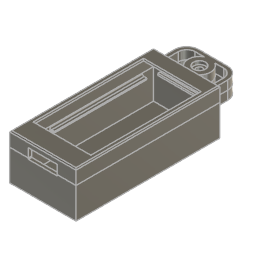
FlightSensorbyLimitens (Autodesk Fusion 360 design; units mm, degrees)
part number: 2026-05-18-21-55-51-119
Autodesk Fusion 360 part; units mm, degrees
sketch "Sketch1" plane through (0, 0, 0) normal (0, 0, 1) x (1, 0, 0)
  line L0 (-1, 32) -> (28, 32)
  line L1 (28, 32) -> (28, -31)
  line L2 (28, -31) -> (-1, -31)
  line L3 (-1, -31) -> (-1, 32)
  line L4 (30, -32) -> (-3, -32)
  line L5 (-3, -32) -> (-3, 34)
  line L6 (-3, 34) -> (30, 34)
  line L7 (30, 34) -> (30, -32)
  line L8 (21, -32) -> (6, -32)
  line L9 (6, -32) -> (6, -31)
  line L10 (6, -31) -> (21, -31)
  line L11 (21, -31) -> (21, -32)
  line L12 (21, -32) -> (6, -31) construction
  line L13 (6, -32) -> (21, -31) construction
  line L14 (19.5, -32) -> (7.5, -32)
  line L15 (7.5, -32) -> (7.5, -31)
  line L16 (7.5, -31) -> (19.5, -31)
  line L17 (19.5, -31) -> (19.5, -32)
  line L18 (19.5, -32) -> (7.5, -31) construction
  line L19 (7.5, -32) -> (19.5, -31) construction
  point P0 (13.5, -31.5)
  point P1 (13.5, -31.5)
  constraint horizontal L0
  constraint vertical L1
  constraint horizontal L2
  constraint vertical L3
  constraint horizontal L4
  constraint vertical L5
  constraint horizontal L6
  constraint vertical L7
  constraint horizontal L8
  constraint perpendicular L8 L9
  constraint parallel L8 L10
  constraint parallel L9 L11
  constraint coincident L12 P1
  constraint coincident L13 P1
  constraint coincident L4 L8.start
  constraint horizontal L14
  constraint perpendicular L14 L15
  constraint parallel L14 L16
  constraint parallel L15 L17
  constraint coincident L18 P1
  constraint coincident L19 P1
  constraint coincident L8 L14.start
  constraint coincident P1 P0
sketch "Sketch2" plane through (7.5, 0, 0) normal (1, 0, 0) x (0, 1, 0)
  line L0 (-33, -3) -> (-33, -5.5)
  line L1 (-33, -5.5) -> (-32, -5.5)
  line L2 (-31, -1.5) -> (-33, -1.5)
  line L3 (-33, -1.5) -> (-33, -5.5)
  line L4 (-33, -5.5) -> (-31, -5.5)
  line L5 (-31, -5.5) -> (-31, -1.5)
  line L6 (-32, -3) -> (-33, -3)
  line L7 (-32, -5.5) -> (-32, -3)
  constraint horizontal L2
  constraint vertical L3
  constraint horizontal L4
  constraint vertical L5
  constraint coincident L0.end L1.start
sketch "Sketch3" plane through (-1, 0, 0) normal (1, 0, 0) x (0, 1, 0)
  line L0 (32, 4) -> (-31, 4)
  line L1 (-31, -3) -> (32, -3)
  line L2 (32, -3) -> (32, 2)
  line L3 (32, 2) -> (-31, 2)
  line L4 (-31, 2) -> (-31, -3)
  line L5 (-31, 3) -> (32, 3)
  line L6 (32, 3) -> (32, 4)
  line L7 (-31, 4) -> (-31, 3)
  constraint horizontal L1
  constraint vertical L2
  constraint horizontal L3
  constraint vertical L4
sketch "Sketch4" plane through (0, 34, 0) normal (0, 1, 0) x (-1, 0, 0)
  line L0 (3, 4) -> (-30, 4)
  line L1 (-2.5, -2.5) -> (-24.5, -2.5)
  line L2 (-24.5, -2.5) -> (-24.5, 1)
  line L3 (-24.5, 1) -> (-2.5, 1)
  line L4 (-2.5, 1) -> (-2.5, -2.5)
  line L5 (-2.5, -2.5) -> (-24.5, 1) construction
  line L6 (-24.5, -2.5) -> (-2.5, 1) construction
  line L7 (3, 3) -> (3, 4)
  line L8 (-30, 4) -> (-30, 3)
  line L9 (-30, 3) -> (3, 3)
  point P0 (-13.5, -0.75)
  constraint horizontal L1
  constraint perpendicular L1 L2
  constraint parallel L1 L3
  constraint parallel L2 L4
  constraint coincident L5 P0
  constraint coincident L6 P0
ref_plane "WorkPlane1" through (13.5, -32, -0.5) normal (0, 0, -1) x (-1, 0, 0)
sketch "Sketch5" plane through (0, 0, 3) normal (0, 0, 1) x (-1, 0, 0)
  circle A0 centre (-13.5, -37.8128) radius 2.75
  arc A1 (-7.5, -42) -> (-2.5, -37) centre (-7.5, -37) ccw
  line L0 (-2.5, -37) -> (-2.5, -34)
  line L1 (-24.5, -34) -> (-24.5, -37)
  arc A2 (-24.5, -37) -> (-19.5, -42) centre (-19.5, -37) ccw
  line L2 (-19.5, -42) -> (-7.5, -42)
  circle A3 centre (-13.5, -37.8128) radius 3.3621
  line L3 (-2.5, -34) -> (-24.5, -34)
  line L4 (-4.3696, -37) -> (-4.3696, -35.8696)
  line L5 (-4.3696, -35.8696) -> (-22.6304, -35.8696)
  line L6 (-22.6304, -35.8696) -> (-22.6304, -37)
  arc A4 (-22.6304, -37) -> (-19.5, -40.1304) centre (-19.5, -37) ccw
  line L7 (-19.5, -40.1304) -> (-7.5, -40.1304)
  arc A5 (-7.5, -40.1304) -> (-4.3696, -37) centre (-7.5, -37) ccw
  dimension "d51" = -1.8696
  dimension "d52" = 0.6121
sketch "Sketch6" plane through (0, -33, 0) normal (0, -1, 0) x (1, 0, 0)
  line L0 (1.4033, -2.2193) -> (8.2394, -2.2193)
  line L1 (8.2394, -2.2193) -> (8.2394, -5.5673)
  line L2 (8.2394, -5.5673) -> (1.4033, -5.5673)
  line L3 (1.4033, -5.5673) -> (1.4033, -2.2193)
  line L4 (-1, 1) -> (28, 1)
  line L5 (28, 1) -> (28, 1.5)
  line L6 (28, 1.5) -> (-1, 1.5)
  line L7 (-1, 1.5) -> (-1, 1)
  constraint horizontal L0
  constraint vertical L1
  constraint horizontal L2
  constraint vertical L3
sketch "Sketch7" plane through (0, 0, 0) normal (0, 0, 1) x (1, 0, 0)
  line L0 (-14, 62) -> (14, 62)
  line L1 (14, 62) -> (14, 0)
  line L2 (14, 0) -> (-14, 0)
  line L3 (-14, 0) -> (-14, 62)
  line L4 (15, -1) -> (-15, -1)
  line L5 (-15, -1) -> (-15, 63)
  line L6 (-15, 63) -> (15, 63)
  line L7 (15, 63) -> (15, -1)
  line L8 (-15, -1) -> (15, -1)
  line L9 (15, -1) -> (15, -2)
  line L10 (15, -2) -> (-15, -2)
  line L11 (-15, -2) -> (-15, -1)
  line L12 (-14, 0) -> (14, 0)
  line L13 (14, 0) -> (14, -0.5)
  line L14 (14, -0.5) -> (-14, -0.5)
  line L15 (-14, -0.5) -> (-14, 0)
  line L16 (6.5, -2) -> (-6.5, -2)
  line L17 (-6.5, -2) -> (-6.5, 1)
  line L18 (-6.5, 1) -> (6.5, 1)
  line L19 (6.5, 1) -> (6.5, -2)
  line L20 (6.5, -2) -> (-6.5, 1) construction
  line L21 (-6.5, -2) -> (6.5, 1) construction
  point P0 (0, -0.5)
  constraint horizontal L0
  constraint vertical L1
  constraint horizontal L2
  constraint vertical L3
  constraint horizontal L4
  constraint vertical L5
  constraint horizontal L6
  constraint vertical L7
  constraint horizontal L8
  constraint vertical L9
  constraint horizontal L10
  constraint vertical L11
  constraint horizontal L12
  constraint vertical L13
  constraint horizontal L14
  constraint vertical L15
  constraint horizontal L16
  constraint perpendicular L16 L17
  constraint parallel L16 L18
  constraint parallel L17 L19
  constraint coincident L20 P0
  constraint coincident L21 P0
  constraint coincident L10 L16.start
  constraint midpoint L14 P0
extrude "Extrude23" add sketch "Sketch7" along normal blind 6.5 contours L0 L1 L3 L4 L5 L6 L7 L8 L13 L14 L15 L17 L19 | L4 L8 L10 L11 L17 | L4 L8 L9 L10 L19 makes body 1
sketch "Sketch8" plane through (0, 0, 6.5) normal (0, 0, 1) x (-1, 0, 0)
  line L0 (6.5, 2) -> (6.5, 0.5)
  line L1 (6.5, 0.5) -> (14, 0.5)
  line L2 (14, 0.5) -> (14, -62)
  line L3 (14, -62) -> (-14, -62)
  line L4 (-14, -62) -> (-14, 0.5)
  line L5 (-14, 0.5) -> (-6.5, 0.5)
  line L6 (-6.5, 0.5) -> (-6.5, 2)
  line L7 (-6.5, 2) -> (-15, 2)
  line L8 (-15, 2) -> (-15, -63)
  line L9 (-15, -63) -> (15, -63)
  line L10 (15, -63) -> (15, 2)
  line L11 (15, 2) -> (6.5, 2)
  line L12 (15, 2) -> (-15, 2)
  line L13 (-15, 2) -> (-15, -63)
  line L14 (-15, -63) -> (15, -63)
  line L15 (15, -63) -> (15, 2)
  line L16 (-13, -6.7) -> (13, -6.7)
  line L17 (13, -6.7) -> (13, -56.5)
  line L18 (13, -56.5) -> (-13, -56.5)
  line L19 (-13, -56.5) -> (-13, -6.7)
  constraint horizontal L12
  constraint vertical L13
  constraint horizontal L14
  constraint vertical L15
  constraint coincident L8.end L9.start
  constraint coincident L10.end L11.start
  constraint horizontal L16
  constraint vertical L17
  constraint horizontal L18
  constraint vertical L19
extrude "Extrude24" cut sketch "Sketch8" against normal blind 1 bodies 1
extrude "Extrude25" add sketch "Sketch8" against normal blind 1 bodies 1
sketch "Sketch9" plane through (0, 0, 5.5) normal (0, 0, -1) x (1, 0, 0)
  line L0 (-6.5, 2) -> (-6.5, 0.5)
  line L1 (-6.5, 0.5) -> (-14, 0.5)
  line L2 (-14, 0.5) -> (-14, -62)
  line L3 (-14, -62) -> (14, -62)
  line L4 (14, -62) -> (14, 0.5)
  line L5 (14, 0.5) -> (6.5, 0.5)
  line L6 (6.5, 0.5) -> (6.5, 2)
  line L7 (6.5, 2) -> (-6.5, 2)
  line L8 (13, -56.5) -> (-13, -56.5)
  line L9 (-13, -56.5) -> (-13, -6.7)
  line L10 (-13, -6.7) -> (13, -6.7)
  line L11 (13, -6.7) -> (13, -56.5)
  line L12 (-6.5, 2) -> (6.5, 2)
  line L13 (6.5, 2) -> (6.5, 0.5)
  line L14 (6.5, 0.5) -> (-6.5, 0.5)
  line L15 (-6.5, 0.5) -> (-6.5, 2)
  constraint horizontal L12
  constraint vertical L13
  constraint horizontal L14
  constraint vertical L15
  constraint coincident L5.end L6.start
  constraint coincident L0.start L7.end
extrude "Extrude26" add sketch "Sketch9" along normal blind 1.5 contours L0 L6 L7 L12 L13 L14 L15 bodies 1
extrude "Extrude27" add 1 faces at (-11.8333, -1.5, 0) along direction (0, 0, -1) blind 8 on bodies 1 bodies 1
extrude "Extrude28" cut 1 faces at (-11.8333, -1.5, -8) along direction (0, 0, 1) blind 1 on bodies 1 bodies 1
sketch "Sketch10" plane through (0, 0, 0) normal (0, 0, 1) x (1, 0, 0)
  line L0 (51, 29) -> (35, 29)
  line L1 (35, 29) -> (35, -17)
  line L2 (35, -17) -> (51, -17)
  line L3 (51, -17) -> (51, 29)
  dimension "d69" = 16
  dimension "d70" = 46
  constraint horizontal L0
  constraint vertical L1
  constraint horizontal L2
  constraint vertical L3
  measures "d69" distance of L0.start L0.end
  measures "d70" distance of L0.start L2.end
sketch "Sketch11" plane through (14, 0, 0) normal (-1, 0, 0) x (0, -1, 0)
  line L0 (-62, -7) -> (0.5, -7)
  line L1 (0.5, -7) -> (0.5, 5.5)
  line L2 (0.5, 5.5) -> (-62, 5.5)
  line L3 (-62, 5.5) -> (-62, -7)
  line L4 (-60.2, -1) -> (-6, -1)
  line L5 (-6, -1) -> (-6, -1.5)
  line L6 (-6, -1.5) -> (-60.2, -1.5)
  line L7 (-60.2, -1.5) -> (-60.2, -1)
  constraint horizontal L4
  constraint vertical L5
  constraint horizontal L6
  constraint vertical L7
extrude "Extrude30" add sketch "Sketch11" along normal blind 2 contours L4 L5 L6 L7 bodies 1
sketch "Sketch12" plane through (0, 62, 0) normal (0, -1, 0) x (1, 0, 0)
  line L0 (-14, -7) -> (14, -7)
  line L1 (14, -7) -> (14, 5.5)
  line L2 (14, 5.5) -> (-14, 5.5)
  line L3 (-14, 5.5) -> (-14, -7)
  line L4 (-11.0417, -0.6543) -> (12.2597, -0.6543)
  line L5 (12.2597, -0.6543) -> (12.2597, -1.4447)
  line L6 (12.2597, -1.4447) -> (-11.0417, -1.4447)
  line L7 (-11.0417, -1.4447) -> (-11.0417, -0.6543)
  constraint horizontal L4
  constraint vertical L5
  constraint horizontal L6
  constraint vertical L7
extrude "Extrude31" add sketch "Sketch12" along normal blind 1 contours L4 L5 L6 L7 bodies 1
sketch "Sketch13" plane through (-14, 0, 0) normal (1, 0, 0) x (0, 1, 0)
  line L0 (-0.5, -7) -> (62, -7)
  line L1 (62, -7) -> (62, 5.5)
  line L2 (62, 5.5) -> (-0.5, 5.5)
  line L3 (-0.5, 5.5) -> (-0.5, -7)
  line L4 (57, -1) -> (15.2249, -1)
  line L5 (15.2249, -1) -> (15.2249, -1.5635)
  line L6 (15.2249, -1.5635) -> (57, -1.5635)
  line L7 (57, -1.5635) -> (57, -1)
  constraint horizontal L4
  constraint vertical L5
  constraint horizontal L6
  constraint vertical L7
extrude "Extrude32" add sketch "Sketch13" along normal blind 1 contours L4 L5 L6 L7 bodies 1
extrude "Extrude33" add 1 faces at (-13, 29.1499, -1.1878) along direction (1, 0, 0) blind 1 on bodies 1 bodies 1
fillet "Fillet3" radius 0.75 1 edges at (-14, 36.1124, -1) on bodies 1
fillet "Fillet4" radius 0.75 1 edges at (14, 33.1, -1) on bodies 1
sketch "Sketch14" plane through (-6.5, 0, 0) normal (1, 0, 0) x (0, 1, 0)
  line L0 (-2, -7) -> (-0.5, -7)
  line L1 (-0.5, -7) -> (-0.5, 4)
  line L2 (-0.5, 4) -> (-2, 4)
  line L3 (-2, 4) -> (-2, -7)
  line L4 (-0.5, -0.5) -> (-2, -0.5)
  line L5 (-2, -0.5) -> (-2, -7)
  line L6 (-2, -7) -> (-0.5, -7)
  line L7 (-0.5, -7) -> (-0.5, -0.5)
  constraint horizontal L4
  constraint vertical L5
  constraint horizontal L6
  constraint vertical L7
  constraint coincident L0.start L3.end
  constraint coincident L1 L4.start
extrude "Extrude34" add sketch "Sketch14" along normal blind 13 contours L0 L1 L3 L4 L5 L6 L7 bodies 1
extrude "Extrude35" add 1 faces at (-4.6667, -1.5, -7) along direction (0, 0, -1) blind 5 on bodies 1 bodies 1
sketch "Sketch15" plane through (0, 63, 0) normal (0, 1, 0) x (-1, 0, 0)
  line L0 (15, -12) -> (15, 6.5)
  line L1 (15, 6.5) -> (-15, 6.5)
  line L2 (-15, 6.5) -> (-15, -12)
  line L3 (-15, -12) -> (15, -12)
  line L4 (12, -4) -> (-12, -4)
  line L5 (-12, -4) -> (-12, 4)
  line L6 (-12, 4) -> (12, 4)
  line L7 (12, 4) -> (12, -4)
  line L8 (12, -4) -> (-12, 4) construction
  line L9 (-12, -4) -> (12, 4) construction
  constraint horizontal L4
  constraint perpendicular L4 L5
  constraint parallel L4 L6
  constraint parallel L5 L7
  constraint coincident L8 origin
  constraint coincident L9 origin
extrude "Extrude36" add sketch "Sketch15" along normal blind 12 contours L4 L5 L6 L7 bodies 1
fillet "Fillet5" radius 5.5 2 edges at (12, 75, 0) (-12, 75, 0) on bodies 1
hole "Hole2" at (0, 68.7747, 4) direction (0, 0, -1) diameter 2.9 depth 7 tip angle 118 counterbore diameter 5.5 counterbore depth 2.5 bodies 1
sketch "Sketch16" plane through (0, 0, 4) normal (0, 0, 1) x (-1, 0, 0)
  circle A0 centre (0, -68.7747) radius 2.75
  arc A1 (6.5, -75) -> (12, -69.5) centre (6.5, -69.5) ccw
  line L0 (12, -69.5) -> (12, -63)
  line L1 (12, -63) -> (-12, -63)
  line L2 (-12, -63) -> (-12, -69.5)
  arc A2 (-12, -69.5) -> (-6.5, -75) centre (-6.5, -69.5) ccw
  line L3 (-6.5, -75) -> (6.5, -75)
  line L4 (10.2578, -64.7422) -> (-10.2578, -64.7422)
  line L5 (-10.2578, -64.7422) -> (-10.2578, -69.5)
  arc A3 (-10.2578, -69.5) -> (-6.5, -73.2578) centre (-6.5, -69.5) ccw
  line L6 (-6.5, -73.2578) -> (6.5, -73.2578)
  arc A4 (6.5, -73.2578) -> (10.2578, -69.5) centre (6.5, -69.5) ccw
  line L7 (10.2578, -69.5) -> (10.2578, -64.7422)
  circle A5 centre (0, -68.7747) radius 5.0983
  dimension "d98" = -1.7422
  dimension "d99" = 2.3483
extrude "Extrude37" cut sketch "Sketch16" against normal blind 16 contours L4 L6 A4 L7 A5 | L4 L5 A3 L6 A5 bodies 1
ref_plane "WorkPlane2" through (0, 30.5, 0) normal (0, 0, -1) x (-1, 0, 0)
split "Split2" by plane through (0, 30.5, 0) normal (0, 0, -1) bodies 1 makes body 2 at (-15, 19.6667, -8)
sketch "Sketch17" plane through (0, 0, -12) normal (0, 0, -1) x (1, 0, 0)
  line L0 (-14, 0.5) -> (14, 0.5)
  line L1 (14, 0.5) -> (14, -62)
  line L2 (14, -62) -> (-14, -62)
  line L3 (-14, -62) -> (-14, 0.5)
  line L4 (15, 2) -> (-15, 2)
  line L5 (-15, 2) -> (-15, -63)
  line L6 (-15, -63) -> (15, -63)
  line L7 (15, -63) -> (15, 2)
  line L8 (15, 2) -> (-15, 2)
  line L9 (-15, 2) -> (-15, -63)
  line L10 (-15, -63) -> (15, -63)
  line L11 (15, -63) -> (15, 2)
  constraint horizontal L8
  constraint vertical L9
  constraint horizontal L10
  constraint vertical L11
  constraint coincident L5.end L6.start
  constraint coincident L4.start L7.end
extrude "Extrude38" cut sketch "Sketch17" against normal blind 1 contours L0 L1 L2 L3 | L4 L5 L6 L7 L8 L9 L10 L11 bodies 2
sketch "Sketch18" plane through (0, 0, -11) normal (0, 0, -1) x (1, 0, 0)
  line L0 (14, 0.5) -> (14, -62)
  line L1 (14, -62) -> (-14, -62)
  line L2 (-14, -62) -> (-14, 0.5)
  line L3 (-14, 0.5) -> (14, 0.5)
  line L4 (15, -63) -> (15, 2)
  line L5 (15, 2) -> (-15, 2)
  line L6 (-15, 2) -> (-15, -63)
  line L7 (-15, -63) -> (15, -63)
  line L8 (-15, -63) -> (15, -63)
  line L9 (15, -63) -> (15, 2)
  line L10 (15, 2) -> (-15, 2)
  line L11 (-15, 2) -> (-15, -63)
  constraint horizontal L8
  constraint vertical L9
  constraint horizontal L10
  constraint vertical L11
  constraint coincident L4.end L5.start
  constraint coincident L6.end L7.start
extrude "Extrude39" add sketch "Sketch18" along normal blind 1 contours L0 L1 L2 L3 | L4 L5 L6 L7 L8 L9 L10 L11 bodies 2
extrude "Extrude40" add 1 faces at (-2.0657, 69.8096, 1.5) along direction (0, 0, 1) blind 1 on bodies 1 bodies 1
extrude "Extrude41" add 1 faces at (-2.0657, 69.8096, 2.5) along direction (0, 0, 1) blind 0.5 on bodies 1 bodies 1
extrude "Extrude42" cut 1 faces at (-2.0657, 69.8096, 3) along direction (0, 0, -1) blind 0.5 on bodies 1 bodies 1
fillet "Fillet7" radius 0.5 tangency weight 0.1 4 edges at (0, -2, 6.5) (15, 30.5, 6.5) (-15, 30.5, 6.5) (0, 63, 6.5) on bodies 1
sketch "Sketch19" plane through (0, 0, 0) normal (0, 0, 1) x (1, 0, 0)
  line L0 (-81, 9) -> (-53, 9)
  line L1 (-53, 9) -> (-53, 58)
  line L2 (-53, 58) -> (-81, 58)
  line L3 (-81, 58) -> (-81, 9)
  dimension "d119" = 28
  dimension "d120" = 49
  constraint horizontal L0
  constraint vertical L1
  constraint horizontal L2
  constraint vertical L3
  measures "d119" distance of L0.start L0.end
  measures "d120" distance of L0.start L2.end
extrude "Extrude44" cut 1 faces at (5, 41.3333, -12) along direction (0, 0, 1) blind 4 on bodies 2 bodies 2
extrude "Extrude45" add 1 faces at (-4.6667, -1.5, -8) along direction (0, 0, -1) blind 5.5 on bodies 2 bodies 2
sketch "Sketch20" plane through (0, 0, -13.5) normal (0, 0, -1) x (1, 0, 0)
  line L0 (-14, -62) -> (-14, 0.5)
  line L1 (-14, 0.5) -> (14, 0.5)
  line L2 (14, 0.5) -> (14, -62)
  line L3 (14, -62) -> (-14, -62)
  line L4 (-15, 2) -> (-15, -63)
  line L5 (-15, -63) -> (15, -63)
  line L6 (15, -63) -> (15, 2)
  line L7 (15, 2) -> (-15, 2)
  line L8 (-15, 2) -> (15, 2)
  line L9 (15, 2) -> (15, -63)
  line L10 (15, -63) -> (-15, -63)
  line L11 (-15, -63) -> (-15, 2)
  constraint horizontal L8
  constraint vertical L9
  constraint horizontal L10
  constraint vertical L11
  constraint coincident L5.end L6.start
  constraint coincident L4.start L7.end
extrude "Extrude46" add sketch "Sketch20" along normal blind 1 contours L0 L1 L2 L3 | L4 L5 L6 L7 L8 L9 L10 L11 bodies 2
extrude "Extrude47" cut 1 faces at (-5, 19.6667, -14.5) along direction (0, 0, 1) blind 1 on bodies 2 bodies 2
extrude "Extrude48" add sketch "Sketch20" along normal blind 1.5 contours L0 L1 L2 L3 | L4 L5 L6 L7 L8 L9 L10 L11 bodies 2
fillet "Fillet9" radius 1 tangency weight 0.1 4 edges at (15, 30.5, -15) (0, -2, -15) (-15, 30.5, -15) (0, 63, -15) on bodies 2
named bodies: "top", "bottom"
